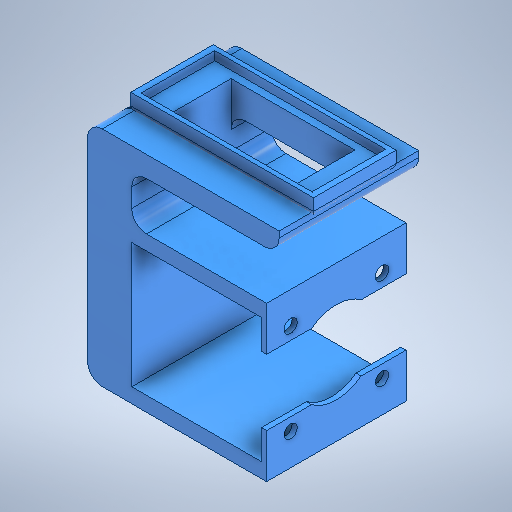
# Autodesk Inventor part: Attache moteur côté rocker
Saved by Autodesk Inventor 2026.2 (Build 302298010, 298A)
## iProperties
Created: 2026-03-22
Part Number: Attache moteur côté rocker
Material: Générique
Document SubType Name: Modeling
Designer: Genon
Density: 1 g/cm^3
Appearance: Cyan
Author: Genon
Autodesk Inventor part; units mm, degrees
sketch "Esquisse1" plane through (0, 0, 0) normal (0, 1, 0) x (-1, 0, 0)
  line L0 (-21, 10.05) -> (21, 10.05)
  line L1 (21, 10.05) -> (21, -10.05)
  line L2 (21, -10.05) -> (-21, -10.05)
  line L3 (-21, -10.05) -> (-21, 10.05)
  line L4 (-21, 10.05) -> (21, -10.05) construction
  line L5 (21, 10.05) -> (-21, -10.05) construction
  line L6 (-29, 12.5) -> (29, 12.5)
  line L7 (29, 12.5) -> (29, -12.5)
  line L8 (29, -12.5) -> (-29, -12.5)
  line L9 (-29, -12.5) -> (-29, 12.5)
  line L10 (-29, 12.5) -> (29, -12.5) construction
  line L11 (29, 12.5) -> (-29, -12.5) construction
  point P0 (0, 0)
  dimension "d0" = 42
  dimension "d1" = 20.1
  dimension "d2" = 58
  dimension "d3" = 25
  constraints: 24 end point, 4 midpoint, 4 parallel, 2 horizontal, 2 perpendicular
  measures "d0" distance of L1.end L2.end
  measures "d1" distance of L0.end L1.end
  measures "d2" distance of L7.end L8.end
  measures "d3" distance of L6.end L7.end
extrude "Extrusion1" add sketch "Esquisse1" along normal blind 10
sketch "Esquisse3" plane through (0, 10, 0) normal (0, 1, 0) x (1, 0, 0)
  line L0 (29, 12.5) -> (-29, 12.5) projected
  line L1 (-29, 12.5) -> (-29, -12.5) projected
  line L2 (-29, -12.5) -> (29, -12.5) projected
  line L3 (29, -12.5) -> (29, 12.5) projected
  line L4 (-31, -14) -> (31, -14)
  line L5 (31, -14) -> (31, 14)
  line L6 (31, 14) -> (-31, 14)
  line L7 (-31, 14) -> (-31, -14)
  line L8 (-31, -14) -> (31, 14) construction
  line L9 (31, -14) -> (-31, 14) construction
  point P0 (0, 0)
  dimension "d12" = 62
  dimension "d13" = 28
  constraints: 12 end point, 2 midpoint, 2 parallel, 1 horizontal, 1 perpendicular
  measures "d12" distance of L6.end L5.end
  measures "d13" distance of L5.end L4.end
extrude "Extrusion3" add sketch "Esquisse3" along normal mid plane 6
fillet "Congé1" radius 2 4 edges at (0, 7, 14) (-31, 7, 0) (0, 7, -14) (31, 7, 0)
sketch "Esquisse4" plane through (-29, 0, -12.5) normal (-1, 0, 0) x (0, 0, 1)
  line L0 (24.5, 7) -> (0.5, 7) projected
  arc A0 (0, 7.0635) -> (0.5, 7) centre (0.5, 9) ccw projected
  line L1 (0, 7.0635) -> (0, 0) projected
  line L2 (0, 0) -> (25, 0) projected
  line L3 (25, 0) -> (25, 7.0635) projected
  arc A1 (24.5, 7) -> (25, 7.0635) centre (24.5, 9) ccw projected
  point P0 (12.5, 0)
extrude "Extrusion4" add sketch "Esquisse4" along normal blind 7
sketch "Esquisse5" plane through (0, 0, 0) normal (0, -1, 0) x (1, 0, 0)
  line L0 (29, 12.5) -> (-36, 12.5) projected
  line L1 (29, -12.5) -> (-36, -12.5) projected
  line L2 (-36, 12.5) -> (-21, 12.5)
  line L3 (-21, 12.5) -> (-21, -12.5)
  line L4 (-21, -12.5) -> (-36, -12.5)
  line L5 (-36, -12.5) -> (-36, 12.5)
  line L6 (0, 0) -> (-21, 0)
  line L7 (-21, 10.05) -> (-21, -10.05) projected
  line L8 (-21, 0) -> (-36, 0)
  line L9 (-36, 0) -> (-36, -12.5)
  line L10 (-36, -12.5) -> (-21, -12.5)
  line L11 (-21, -12.5) -> (-21, 12.5)
  line L12 (-21, 12.5) -> (-36, 12.5)
  line L13 (-36, 12.5) -> (-36, 0)
  dimension "d19" = 15
  dimension "d85" = 15
  constraints: 22 end point, 7 point on line, 4 perpendicular, 2 parallel, 1 horizontal, 1 midpoint
  measures "d19" distance of L3.end L4.end
  measures "d85" distance of L6.end L8.end
extrude "Extrusion5" add sketch "Esquisse5" along normal blind 42.5
fillet "Congé2" radius 5 3 edges at (-36, 7.0159, -12.252) (-36, 7.0159, 12.252) (-36, 7, 0)
fillet "Congé3" radius 5 1 edges at (29, 0, 0)
sketch "Esquisse6" plane through (0, -42.5, 0) normal (0, -1, 0) x (1, 0, 0)
  line L0 (-36, -12.5) -> (-21, -12.5) projected
  line L1 (-21, 12.5) -> (-36, 12.5) projected
  line L2 (-21, -12.5) -> (-21, 12.5) projected
  line L3 (-36, 12.5) -> (-36, -12.5) projected
  point P0 (0, 0)
extrude "Extrusion6" add sketch "Esquisse6" along normal blind 21.15
ref_plane "Plan de construction1" through (0, -42.5, 0) normal (0, 1, 0) x (-1, 0, 0)
sketch "Esquisse7" plane through (0, -63.65, 0) normal (0, -1, 0) x (1, 0, 0)
  line L0 (-21, 12.5) -> (-36, 12.5) projected
  line L1 (-36, -12.5) -> (-21, -12.5) projected
  line L2 (-21, -12.5) -> (-21, 12.5) projected
  line L3 (-36, 12.5) -> (-36, -12.5) projected
  point P0 (0, 0)
extrude "Extrusion7" add sketch "Esquisse7" along normal blind 5
ref_plane "Plan de construction3" through (0, -21.3, 0) normal (0, 1, 0) x (-1, 0, 0)
ref_plane "Plan de construction4" through (0, -63.7, 0) normal (0, 1, 0) x (-1, 0, 0)
sketch "Esquisse10" plane through (0, -63.7, 0) normal (0, 1, 0) x (-1, 0, 0)
  line L0 (-23, -12.5) -> (-23, 12.5)
  line L1 (21, -12.5) -> (21, 12.5) projected
  line L2 (21, -12.5) -> (-23, -12.5)
  line L3 (21, 12.5) -> (-23, 12.5)
  point P0 (0, 0)
  point P1 (36, 12.5)
  constraints: 6 end point, 1 parallel, 1 perpendicular
extrude "Extrusion10" add sketch "Esquisse10" against normal blind 5
sketch "Esquisse11" plane through (0, -63.7, 0) normal (0, 1, 0) x (-1, 0, 0)
  line L0 (36, -12.5) -> (-23, -12.5) projected
  line L1 (-23, -12.5) -> (-24.75, -12.5)
  line L2 (-24.75, -12.5) -> (-24.75, 12.5)
  line L3 (-24.75, 12.5) -> (-23, 12.5)
  line L4 (-23, 12.5) -> (-23, -12.5)
  point P0 (0, 0)
  point P1 (39, -12.5)
  dimension "d41" = 1.75
  dimension "d42" = 25
  constraints: 8 end point, 2 parallel, 1 horizontal, 1 perpendicular
  measures "d41" distance of L2.end L3.end
  measures "d42" distance of L1.end L2.end
sketch "Esquisse12" plane through (23, -63.7, 12.5) normal (1, 0, 0) x (0, 0, -1)
  line L0 (0, 0) -> (25, 0) projected
  line L1 (0, 0) -> (0, -5) projected
  line L2 (25, -5) -> (0, -5) projected
  line L3 (25, 0) -> (25, -5) projected
  point P0 (12.5, 63.7)
extrude "Extrusion11" add sketch "Esquisse12" along normal blind 1.75
extrude "Extrusion12" add sketch "Esquisse11" along normal blind 10
sketch "Esquisse13" plane through (0, -21.3, 0) normal (0, 1, 0) x (-1, 0, 0)
  line L0 (-23, 12.5) -> (-23, -12.5) projected
  line L1 (-23, -12.5) -> (21, -12.5) projected
  line L2 (21, 12.5) -> (-23, 12.5) projected
  line L3 (21, 12.5) -> (21, -12.5) projected
  point P0 (0, 0)
extrude "Extrusion13" add sketch "Esquisse13" along normal blind 5
sketch "Esquisse14" plane through (23, -21.3, 12.5) normal (1, 0, 0) x (0, 0, -1)
  line L0 (0, 0) -> (25, 0) projected
  line L1 (25, 0) -> (25, 5) projected
  line L2 (0, 5) -> (25, 5) projected
  line L3 (0, 0) -> (0, 5) projected
  point P0 (12.5, 21.3)
extrude "Extrusion14" add sketch "Esquisse14" along normal blind 1.75
sketch "Esquisse15" plane through (0, -21.3, 0) normal (0, -1, 0) x (1, 0, 0)
  line L0 (-21, 12.5) -> (24.75, 12.5) projected
  line L1 (-21, -12.5) -> (24.75, -12.5) projected
  line L2 (24.75, 12.5) -> (23, 12.5)
  line L3 (23, 12.5) -> (23, -12.5)
  line L4 (23, -12.5) -> (24.75, -12.5)
  line L5 (24.75, -12.5) -> (24.75, 12.5)
  point P0 (0, 0)
  point P1 (-34, 12.5)
  point P2 (-34, -12.5)
  point P3 (24.75, -12.5)
  dimension "d52" = 1.75
  constraints: 8 end point, 2 parallel, 1 horizontal, 1 perpendicular, 1 point on line
  measures "d52" distance of L4.end L3.end
extrude "Extrusion15" add sketch "Esquisse15" along normal blind 10
sketch "Esquisse17" plane through (-29.5, 7.0635, 12.5) normal (0, 0, 1) x (1, 0, 0)
  line L0 (52.5, -28.3635) -> (52.5, -38.3635) projected
  line L1 (54.25, -38.3635) -> (52.5, -38.3635) projected
  line L2 (54.25, -23.3635) -> (54.25, -38.3635) projected
  arc A0 (53.5, -7.0635) -> (58.5, -2.0635) centre (53.5, -2.0635) ccw projected
  line L3 (58.5, -2.0635) -> (58.5, 0) projected
  line L4 (0, 0) -> (58.5, 0) projected
  line L5 (0, 0) -> (-1.5, 0) projected
  spline S0 degree 6 poles (-6.5, -5.0456) (-6.5, -4.7068) (-6.4726, -4.3679) (-6.4178, -4.0318) (-6.336, -3.7013) (-6.228, -3.3789) (-5.9561, -2.7418) (-5.7898, -2.428) (-5.5974, -2.1288) (-5.3807, -1.8467) (-5.1417, -1.5842) (-4.7649, -1.2341) (-4.6432, -1.1293) (-4.5175, -1.0292) (-4.3881, -0.9339) (-4.2553, -0.8436) (-4.0724, -0.7292) (-4.0252, -0.7005) (-3.9776, -0.6724) (-3.9297, -0.645) (-3.8814, -0.6182) (-3.7691, -0.5578) (-3.7049, -0.5247) (-3.64, -0.4927) (-3.5747, -0.4618) (-3.5088, -0.432) (-3.352, -0.3644) (-3.2607, -0.3276) (-3.1685, -0.2929) (-3.0756, -0.2604) (-2.9818, -0.2302) (-2.6627, -0.1355) (-2.4341, -0.0816) (-2.2026, -0.0409) (-1.9691, -0.0136) (-1.7345, 0) (-1.5, 0) knots 0 0 0 0 0 0 0 0.257896 0.257896 0.257896 0.257896 0.257896 0.52724 0.52724 0.52724 0.52724 0.52724 0.649449 0.649449 0.649449 0.649449 0.649449 0.691501 0.691501 0.691501 0.691501 0.691501 0.746535 0.746535 0.746535 0.746535 0.746535 0.821498 0.821498 0.821498 0.821498 0.821498 1 1 1 1 1 1 1 projected
  line L6 (8.5, -7.0635) -> (8.5, -23.3635) projected
  line L7 (53.5, -7.0635) -> (8.5, -7.0635) projected
  line L8 (-6.5, -5.0456) -> (-6.5, -75.7135) projected
  line L9 (8.5, -23.3635) -> (54.25, -23.3635) projected
  line L10 (8.5, -28.3635) -> (52.5, -28.3635) projected
  line L11 (8.5, -28.3635) -> (8.5, -70.7635) projected
  line L12 (8.5, -75.7635) -> (54.25, -75.7635) projected
  line L13 (54.25, -75.7635) -> (54.25, -60.7635) projected
  line L14 (52.5, -60.7635) -> (54.25, -60.7635) projected
  line L15 (52.5, -70.7635) -> (52.5, -60.7635) projected
  line L16 (8.5, -70.7635) -> (52.5, -70.7635) projected
  line L17 (8.5, -75.7135) -> (-6.5, -75.7135) projected
  line L18 (8.5, -75.7135) -> (8.5, -75.7635) projected
  point P0 (29.5, -7.0635)
  constraints: 1 other
extrude "Extrusion16" add sketch "Esquisse17" along normal blind 11.15
sketch "Esquisse18" plane through (29, 7.0635, -12.5) normal (0, 0, -1) x (-1, 0, 0)
  line L0 (65, -5.0456) -> (65, -75.7135) projected
  spline S0 degree 6 poles (60, 0) (60.2345, 0) (60.4691, -0.0136) (60.7026, -0.0409) (60.9341, -0.0816) (61.1627, -0.1355) (61.4818, -0.2302) (61.5756, -0.2604) (61.6685, -0.2929) (61.7607, -0.3276) (61.852, -0.3644) (62.0088, -0.432) (62.0747, -0.4618) (62.14, -0.4927) (62.2049, -0.5247) (62.2691, -0.5578) (62.3814, -0.6182) (62.4297, -0.645) (62.4776, -0.6724) (62.5252, -0.7005) (62.5724, -0.7292) (62.7553, -0.8436) (62.8881, -0.9339) (63.0175, -1.0292) (63.1432, -1.1293) (63.2649, -1.2341) (63.6417, -1.5842) (63.8807, -1.8467) (64.0974, -2.1288) (64.2898, -2.428) (64.4561, -2.7418) (64.728, -3.3789) (64.836, -3.7013) (64.9178, -4.0318) (64.9726, -4.3679) (65, -4.7068) (65, -5.0456) knots 0 0 0 0 0 0 0 0.178502 0.178502 0.178502 0.178502 0.178502 0.253465 0.253465 0.253465 0.253465 0.253465 0.308499 0.308499 0.308499 0.308499 0.308499 0.350551 0.350551 0.350551 0.350551 0.350551 0.47276 0.47276 0.47276 0.47276 0.47276 0.742104 0.742104 0.742104 0.742104 0.742104 1 1 1 1 1 1 1 projected
  line L1 (58.5, 0) -> (60, 0) projected
  line L2 (58.5, 0) -> (0, 0) projected
  line L3 (0, 0) -> (0, -2.0635) projected
  arc A0 (0, -2.0635) -> (5, -7.0635) centre (5, -2.0635) ccw projected
  line L4 (50, -23.3635) -> (4.25, -23.3635) projected
  line L5 (4.25, -23.3635) -> (4.25, -38.3635) projected
  line L6 (6, -38.3635) -> (4.25, -38.3635) projected
  line L7 (6, -28.3635) -> (6, -38.3635) projected
  line L8 (50, -28.3635) -> (6, -28.3635) projected
  line L9 (5, -7.0635) -> (50, -7.0635) projected
  line L10 (50, -7.0635) -> (50, -23.3635) projected
  line L11 (50, -28.3635) -> (50, -70.7635) projected
  line L12 (6, -70.7635) -> (50, -70.7635) projected
  line L13 (6, -70.7635) -> (6, -60.7635) projected
  line L14 (4.25, -60.7635) -> (6, -60.7635) projected
  line L15 (4.25, -75.7635) -> (4.25, -60.7635) projected
  line L16 (50, -75.7635) -> (4.25, -75.7635) projected
  line L17 (50, -75.7135) -> (50, -75.7635) projected
  line L18 (65, -75.7135) -> (50, -75.7135) projected
  point P0 (29, -7.0635)
  constraints: 1 other
extrude "Extrusion17" add sketch "Esquisse18" along normal blind 11.15
fillet "Congé6" radius 5 1 edges at (-36, -68.65, 0)
fillet "Congé7" radius 5 3 edges at (-21, -16.3, 0) (-21, 0, 16.85) (-21, 0, -16.85)
sketch "Esquisse23" plane through (24.75, -21.3, 12.5) normal (1, 0, 0) x (0, 0, -1)
  point P0 (12.5, 21.3)
sketch "Esquisse24" plane through (24.75, -21.3, 12.5) normal (1, 0, 0) x (0, 0, -1)
  point P0 (12.5, 21.3)
ref_plane "Plan de construction9" through (24.75, -63.7, 23.65) normal (1, 0, 0) x (0, 0, -1)
ref_plane "Plan de construction10" through (0, -42.5, 0) normal (0, 1, 0) x (1, 0, 0)
sketch "Esquisse26" plane through (24.75, -63.7, 23.65) normal (1, 0, 0) x (0, 0, -1)
  line L0 (0, 0) -> (0, 42.4) projected
  line L1 (47.3, 42.4) -> (47.3, 0) projected
  line L2 (0, 21.2) -> (47.3, 21.2)
  line L3 (23.65, 21.2) -> (23.65, 36.7)
  line L4 (23.65, 36.7) -> (39.15, 36.7)
  line L5 (23.65, 36.7) -> (8.15, 36.7)
  point P0 (23.65, 63.7)
  point P1 (39.15, 5.7)
  point P2 (8.15, 5.7)
  dimension "d93" = 15.5
  dimension "d94" = 15.5
  dimension "d95" = 15.5
  constraints: 8 end point, 3 midpoint, 2 coincident, 2 symmetric about line, 1 horizontal, 1 perpendicular, 1 vertical
  measures "d93" distance of L3.start L3.end
  measures "d94" distance of L3.end L4.end
  measures "d95" distance of L3.end L5.end
hole "Perçage2" at (24.75, -27, 15.5) at (24.75, -27, -15.5) at (24.75, -58, -15.5) at (24.75, -58, 15.5) direction (-1, 0, 0) diameter 4.5 depth 8 tip angle 118
sketch "Esquisse27" plane through (24.75, -21.3, 12.5) normal (1, 0, 0) x (0, 0, -1)
  point P0 (12.5, 21.3)
sketch "Esquisse28" plane through (24.75, -63.7, 23.65) normal (1, 0, 0) x (0, 0, -1)
  line L0 (0, 32.4) -> (47.3, 32.4) projected
  line L1 (47.3, 10) -> (0, 10) projected
  line L2 (23.65, 10) -> (23.65, 32.4)
  circle A0 centre (23.65, 21.2) radius 11
  circle A1 centre (23.65, 21.2) radius 14
  point P0 (23.65, 63.7)
  point P1 (15.25, 10)
  point P2 (32.05, 10)
  point P3 (32.05, 32.4)
  point P4 (15.25, 32.4)
  dimension "d103" = 22
  dimension "d104" = 28
  constraints: 3 midpoint, 2 centre point, 2 end point, 1 coincident
  measures "d103" diameter of A0
  measures "d104" diameter of A1
extrude "Extrusion21" cut sketch "Esquisse28" against normal blind 5 contours A1 L0 | L1 A1
